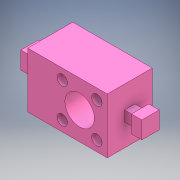
# Autodesk Inventor part: capuchon_roulement
Saved by Autodesk Inventor 2019 (Build 230136000, 136)
## iProperties
Created: 2017-12-27
Part Number: capuchon_roulement
Material: Generic
Document SubType Name: Modeling
Designer: franc
Density: 1 g/cm^3
Appearance: Default
Mass: 2.33274 g
Surface Area: 21.7574 cm^2
Volume: 2.33274 cm^3
Author: franc
Autodesk Inventor part; units mm, degrees
ref_plane "YZ Plane" through (0, 0, 0) normal (1, 0, 0) x (0, 1, 0)
ref_plane "XZ Plane" through (0, 0, 0) normal (0, 1, 0) x (-1, 0, 0)
ref_plane "XY Plane" through (0, 0, 0) normal (0, 0, 1) x (1, 0, 0)
sketch "Esquisse1" plane through (0, 0, 0) normal (0, 1, 0) x (-1, 0, 0)
  line L0 (4.4286, 5.3714) -> (-11.5714, 5.3714)
  line L1 (-11.5714, 5.3714) -> (-11.5714, -10.6286)
  line L2 (-11.5714, -10.6286) -> (4.4286, -10.6286)
  line L3 (4.4286, -10.6286) -> (4.4286, 5.3714)
  point P0 (0, 0)
  dimension "d0" = 16
  dimension "d1" = 16
  constraints: 8 end point, 2 parallel, 1 horizontal, 1 perpendicular
  measures "d0" distance of L2.end L0.start
  measures "d1" distance of L0.start L0.end
extrude "Extrusion1" add sketch "Esquisse1" along normal blind 13
sketch "Esquisse2" plane through (0, 0, 0) normal (0, -1, 0) x (1, 0, 0)
  circle A0 centre (3.5714, -2.6286) radius 4.25
  line L0 (-4.4286, 5.3714) -> (11.5714, 5.3714) projected
  line L1 (11.5714, 5.3714) -> (11.5714, -10.6286) projected
  point P0 (0, 0)
  dimension "d4" = 8
  dimension "d5" = 8
  dimension "d6" = 8.5
  constraints: 1 centre point
  measures "d4" distance from line of L0 A0.centre
  measures "d5" distance from line of L1 A0.centre
  measures "d6" diameter of A0
extrude "Extrusion2" cut sketch "Esquisse2" against normal blind 12
sketch "Esquisse3" plane through (3.5714, 12, -2.6286) normal (0, -1, 0) x (1, 0, 0)
  circle A0 centre (0, 0) radius 2.75
  line L0 (8, -8) -> (-8, -8) projected
  line L1 (8, 8) -> (8, -8) projected
  point P0 (-3.5714, 2.6286)
  dimension "d9" = 5.5
  dimension "d10" = 8
  dimension "d11" = 8
  constraints: 1 centre point
  measures "d9" diameter of A0
  measures "d10" distance from line of L0 A0.centre
  measures "d11" distance from line of L1 A0.centre
extrude "Extrusion3" cut sketch "Esquisse3" against normal through all
sketch "Esquisse4" plane through (0, 0, 0) normal (0, -1, 0) x (1, 0, 0)
  circle A0 centre (8.5714, 2.3714) radius 1.5
  circle A1 centre (-1.4286, 2.3714) radius 1.5
  circle A2 centre (-1.4286, -7.6286) radius 1.5
  circle A3 centre (8.5714, -7.6286) radius 1.5
  line L0 (-4.4286, -10.6286) -> (-4.4286, 5.3714) projected
  line L1 (-4.4286, 5.3714) -> (11.5714, 5.3714) projected
  line L2 (11.5714, 5.3714) -> (11.5714, -10.6286) projected
  line L3 (11.5714, -10.6286) -> (-4.4286, -10.6286) projected
  point P0 (0, 0)
  dimension "d14" = 3
  dimension "d15" = 3
  dimension "d16" = 3
  dimension "d17" = 3
  dimension "d19" = 3
  dimension "d20" = 3
  dimension "d21" = 3
  dimension "d22" = 3
  dimension "d23" = 3
  dimension "d24" = 3
  dimension "d25" = 3
  dimension "d26" = 3
  constraints: 4 centre point
  measures "d14" diameter of A0
  measures "d15" diameter of A3
  measures "d16" diameter of A2
  measures "d17" diameter of A1
  measures "d19" distance from line of L1 A0.centre
  measures "d20" distance from line of L2 A0.centre
  measures "d21" distance from line of L2 A3.centre
  measures "d22" distance from line of L3 A3.centre
  measures "d23" distance from line of L3 A2.centre
  measures "d24" distance from line of L0 A2.centre
  measures "d25" distance from line of L0 A1.centre
  measures "d26" distance from line of L1 A1.centre
extrude "Extrusion4" cut sketch "Esquisse4" against normal through all contours A0 | A1 | A2 | A3
sketch "Esquisse6" plane through (11.5714, 0, 5.3714) normal (1, 0, 0) x (0, 0, -1)
  line L0 (6.5, 8) -> (9.5, 8)
  line L1 (9.5, 8) -> (9.5, 5)
  line L2 (9.5, 5) -> (6.5, 5)
  line L3 (6.5, 5) -> (6.5, 8)
  line L4 (0, 0) -> (0, 13) projected
  line L5 (0, 13) -> (16, 13) projected
  point P0 (5.3714, 0)
  dimension "d29" = 3
  dimension "d30" = 3
  dimension "d31" = 6.5
  dimension "d32" = 5
  constraints: 8 end point, 2 parallel, 1 horizontal, 1 perpendicular
  measures "d29" distance of L0.start L0.end
  measures "d30" distance of L2.end L0.start
  measures "d31" distance between parallel lines of L4 L3
  measures "d32" distance between parallel lines of L5 L0
extrude "Extrusion5" add sketch "Esquisse6" along normal blind 3
sketch "Esquisse7" plane through (14.5714, 0, 5.3714) normal (1, 0, 0) x (0, 0, -1)
  line L0 (5.5, 9) -> (10.5, 9)
  line L1 (10.5, 9) -> (10.5, 4)
  line L2 (10.5, 4) -> (5.5, 4)
  line L3 (5.5, 4) -> (5.5, 9)
  line L4 (0, 13) -> (16, 13) projected
  line L5 (0, 0) -> (0, 13) projected
  point P0 (5.3714, 0)
  dimension "d35" = 5
  dimension "d36" = 5
  dimension "d37" = 4
  dimension "d38" = 5.5
  constraints: 8 end point, 2 parallel, 1 horizontal, 1 perpendicular
  measures "d35" distance of L2.end L0.start
  measures "d36" distance of L0.start L0.end
  measures "d37" distance between parallel lines of L4 L0
  measures "d38" distance between parallel lines of L5 L3
extrude "Extrusion6" add sketch "Esquisse7" along normal blind 3
sketch "Esquisse8" plane through (-4.4286, 0, -10.6286) normal (-1, 0, 0) x (0, 0, 1)
  line L0 (0, 0) -> (0, 13) projected
  line L1 (0, 13) -> (16, 13)
  line L2 (16, 13) -> (16, 0)
  line L3 (16, 0) -> (0, 0)
  line L4 (0, 0) -> (0, 13)
  point P0 (10.6286, 0)
  constraints: 8 end point, 2 parallel, 1 horizontal, 1 perpendicular
extrude "Extrusion7" add sketch "Esquisse8" along normal blind 7
sketch "Esquisse9" plane through (-11.4286, 0, -10.6286) normal (-1, 0, 0) x (0, 0, 1)
  line L0 (9.5, 8) -> (6.5, 8)
  line L1 (6.5, 8) -> (6.5, 5)
  line L2 (6.5, 5) -> (9.5, 5)
  line L3 (9.5, 5) -> (9.5, 8)
  line L4 (16, 0) -> (16, 13) projected
  line L5 (16, 13) -> (0, 13) projected
  point P0 (10.6286, 0)
  dimension "d43" = 6.5
  dimension "d44" = 5
  dimension "d45" = 3
  dimension "d46" = 3
  constraints: 8 end point, 2 parallel, 1 horizontal, 1 perpendicular
  measures "d43" distance between parallel lines of L4 L3
  measures "d44" distance between parallel lines of L5 L0
  measures "d45" distance of L2.end L0.start
  measures "d46" distance of L1.end L2.end
extrude "Extrusion8" add sketch "Esquisse9" along normal blind 3
sketch "Esquisse10" plane through (-14.4286, 0, -10.6286) normal (-1, 0, 0) x (0, 0, 1)
  line L0 (10.5, 9) -> (5.5, 9)
  line L1 (5.5, 9) -> (5.5, 4)
  line L2 (5.5, 4) -> (10.5, 4)
  line L3 (10.5, 4) -> (10.5, 9)
  line L4 (16, 0) -> (16, 13) projected
  line L5 (0, 0) -> (16, 0) projected
  point P0 (10.6286, 0)
  dimension "d49" = 5.5
  dimension "d50" = 4
  dimension "d51" = 5
  dimension "d52" = 5
  constraints: 8 end point, 2 parallel, 1 horizontal, 1 perpendicular
  measures "d49" distance between parallel lines of L4 L3
  measures "d50" distance between parallel lines of L5 L2
  measures "d51" distance of L2.end L0.start
  measures "d52" distance of L0.start L0.end
extrude "Extrusion9" add sketch "Esquisse10" along normal blind 3
